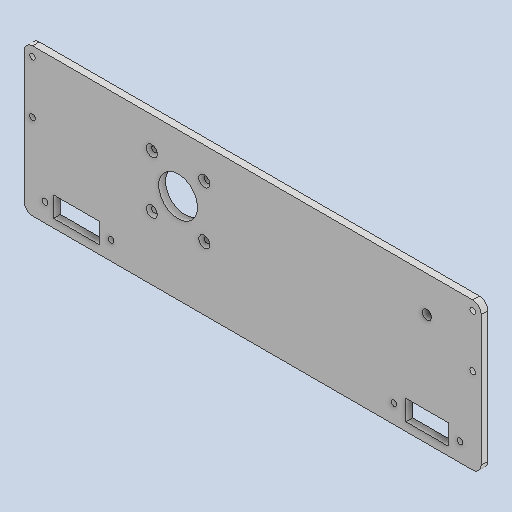
# Autodesk Inventor part: plate_2
Saved by Autodesk Inventor 2024 (Build 280153000, 153)
## iProperties
Created: 2026-02-04
Part Number: plate_2
Material: Generic
Document SubType Name: Modeling
Designer: SEMEN
Density: 1 g/cm^3
Appearance: Default
Author: SEMEN
Autodesk Inventor part; units mm, degrees
ref_plane "YZ Plane" through (0, 0, 0) normal (1, 0, 0) x (0, 1, 0)
ref_plane "XZ Plane" through (0, 0, 0) normal (0, 1, 0) x (-1, 0, 0)
ref_plane "XY Plane" through (0, 0, 0) normal (0, 0, 1) x (1, 0, 0)
sketch "Sketch1" plane through (0, 0, 0) normal (0, 0, 1) x (1, 0, 0)
  arc A0 (235.6827, -57.867) -> (240.6827, -52.867) centre (235.6827, -52.867) ccw projected
  line L0 (240.6827, -52.867) -> (240.6827, 24.133) projected
  arc A1 (240.6827, 24.133) -> (235.6827, 29.133) centre (235.6827, 24.133) ccw projected
  line L1 (235.6827, 29.133) -> (-24.3173, 29.133) projected
  arc A2 (-24.3173, 29.133) -> (-29.3173, 24.133) centre (-24.3173, 24.133) ccw projected
  line L2 (-29.3173, 24.133) -> (-29.3173, -52.867) projected
  arc A3 (-29.3173, -52.867) -> (-24.3173, -57.867) centre (-24.3173, -52.867) ccw projected
  line L3 (-24.3173, -57.867) -> (235.6827, -57.867) projected
  circle A4 centre (235.6827, 23.633) radius 1.7 projected
  circle A5 centre (235.6827, -7.367) radius 1.7 projected
  circle A6 centre (-24.3173, -7.367) radius 1.7 projected
  circle A7 centre (-24.3173, 23.633) radius 1.7 projected
  circle A8 centre (208.6827, 8.133) radius 2.75 projected
  circle A9 centre (228.1827, -46.867) radius 3.3 projected
  circle A10 centre (189.1827, -46.867) radius 3.3 projected
  circle A11 centre (22.1827, -46.867) radius 3.3 projected
  circle A12 centre (-16.8173, -46.867) radius 3.3 projected
  circle A13 centre (235.6827, -7.367) radius 1.7 projected
  circle A14 centre (235.6827, 23.633) radius 1.7 projected
  circle A15 centre (-24.3173, 23.633) radius 1.7 projected
  circle A16 centre (-24.3173, -7.367) radius 1.7 projected
  arc A17 (235.6827, -57.867) -> (240.6827, -52.867) centre (235.6827, -52.867) ccw projected
  line L4 (240.6827, -52.867) -> (240.6827, 24.133) projected
  arc A18 (240.6827, 24.133) -> (235.6827, 29.133) centre (235.6827, 24.133) ccw projected
  line L5 (235.6827, 29.133) -> (-24.3173, 29.133) projected
  arc A19 (-24.3173, 29.133) -> (-29.3173, 24.133) centre (-24.3173, 24.133) ccw projected
  line L6 (-29.3173, 24.133) -> (-29.3173, -52.867) projected
  arc A20 (-29.3173, -52.867) -> (-24.3173, -57.867) centre (-24.3173, -52.867) ccw projected
  line L7 (-24.3173, -57.867) -> (235.6827, -57.867) projected
  circle A21 centre (17.1827, -7.367) radius 3.3 projected
  circle A22 centre (17.1827, 23.633) radius 3.3 projected
  circle A23 centre (-13.8173, 23.633) radius 3.3 projected
  circle A24 centre (-13.8173, -7.367) radius 3.3 projected
  circle A25 centre (208.6827, 8.133) radius 2.75 projected
  circle A26 centre (1.6827, 8.133) radius 11.5 projected
  line L8 (221.1827, -40.867) -> (221.1827, -52.867) projected
  line L9 (221.1827, -52.867) -> (196.1827, -52.867) projected
  line L10 (196.1827, -52.867) -> (196.1827, -40.867) projected
  line L11 (196.1827, -40.867) -> (221.1827, -40.867) projected
  line L12 (-11.8173, -52.867) -> (-11.8173, -40.867) projected
  line L13 (-11.8173, -40.867) -> (15.1827, -40.867) projected
  line L14 (15.1827, -40.867) -> (15.1827, -52.867) projected
  line L15 (15.1827, -52.867) -> (-11.8173, -52.867) projected
extrude "Extrusion1" add sketch "Sketch1" along normal blind 4 contours L3 A3 L2 A2 L1 A1 L0 A0 | A4 | A5 | A6 | A7 | A8 | A9 | A10 | A11 | A12 | A21 | A22 | A23 | A24 | A26
hole "Hole1" at (-24.3173, -7.367, 0) at (-24.3173, 23.633, 0) at (235.6827, 23.633, 0) at (235.6827, -7.367, 0) direction (0, 0, 1) diameter 3.4 end through all clearance for "Countersunk Head GOST 12876-67" size "M3" standard "GOST"
hole "Hole2" at (208.6827, 8.133, 0) direction (0, 0, 1) diameter 5.5 end through all clearance for "Countersunk Head GOST 12876-67" size "M5" standard "GOST"
hole "Hole3" at (-16.8173, -46.867, 0) at (22.1827, -46.867, 0) at (189.1827, -46.867, 0) at (228.1827, -46.867, 0) direction (0, 0, 1) diameter 3.4 end through all countersink diameter 6.6 countersink angle 90 clearance for "Countersunk Head GOST 12876-67" size "M3" standard "GOST"
sketch "Sketch2" plane through (0, 0, 4) normal (0, 0, 1) x (1, 0, 0)
  circle A0 centre (77.1816, -20.3196) radius 1.7 projected
  circle A1 centre (77.1816, 10.6804) radius 1.7 projected
  circle A2 centre (46.1816, 10.6804) radius 1.7 projected
  circle A3 centre (46.1816, -20.3196) radius 1.7 projected
  circle A4 centre (61.6816, -4.8196) radius 11 projected
  line L0 (79.1816, 16.1804) -> (82.6816, 12.6804) projected
  line L1 (79.1816, 16.1804) -> (44.1816, 16.1804) projected
  line L2 (40.6816, 12.6804) -> (44.1816, 16.1804) projected
  line L3 (40.6816, 12.6804) -> (40.6816, -22.3196) projected
  line L4 (44.1816, -25.8196) -> (40.6816, -22.3196) projected
  line L5 (44.1816, -25.8196) -> (79.1816, -25.8196) projected
  line L6 (82.6816, -22.3196) -> (79.1816, -25.8196) projected
  line L7 (82.6816, -22.3196) -> (82.6816, 12.6804) projected
  circle A5 centre (61.6816, -4.8196) radius 11.5
  point P0 (0, 0)
  dimension "d23" = 0.5
  constraints: 1 centre point
  measures "d23" radial gap between concentric circles of A4 A5
extrude "Extrusion2" cut sketch "Sketch2" against normal through all contours A4 | A5
hole "Hole4" at (46.1816, -20.3196, 4) at (46.1816, 10.6804, 4) at (77.1816, 10.6804, 4) at (77.1816, -20.3196, 4) direction (0, 0, -1) diameter 3.4 end through all countersink diameter 6.6 countersink angle 90 clearance for "Countersunk Head GOST 12876-67" size "M3" standard "GOST"
body "Solid1"
